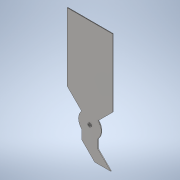
# Autodesk Inventor part: leftside0
Saved by Autodesk Inventor 2020 (Build 240168000, 168)
## iProperties
Created: 2020-04-30
Part Number: leftside0
Material: Generic
Document SubType Name: Modeling
Designer: LENOVO
Density: 1 g/cm^3
Appearance: Default
Author: LENOVO
Autodesk Inventor part; units mm, degrees
ref_plane "YZ Plane" through (0, 0, 0) normal (1, 0, 0) x (0, 1, 0)
ref_plane "XZ Plane" through (0, 0, 0) normal (0, 1, 0) x (-1, 0, 0)
ref_plane "XY Plane" through (0, 0, 0) normal (0, 0, 1) x (1, 0, 0)
sketch "Sketch1" plane through (0, 0, 0) normal (0, 0, 1) x (1, 0, 0)
  line L0 (-100, 150) -> (100, 150)
  line L1 (100, 150) -> (100, -150)
  line L2 (-100, -150) -> (-100, 150)
  line L3 (-100, 150) -> (100, -150) construction
  line L4 (100, 150) -> (-100, -150) construction
  line L5 (100, -150) -> (36.4382, -213.5618)
  line L6 (-35.3571, -283.1536) -> (-35.3571, -323.1554)
  line L7 (-35.3571, -323.1554) -> (21.2114, -379.7239)
  line L8 (35.3571, -283.1536) -> (35.3571, -323.1554)
  line L9 (35.3571, -323.1554) -> (91.9257, -379.7239)
  line L10 (91.9257, -379.7239) -> (21.2114, -379.7239)
  arc A0 (-35.3571, -283.1536) -> (-35.3553, -283.1554) centre (0, -247.8) ccw
  arc A1 (-36.4382, -213.5618) -> (-35.3553, -283.1554) centre (0, -247.8) ccw
  arc A2 (35.3571, -283.1536) -> (36.4382, -213.5618) centre (0, -247.8) ccw
  line L11 (-100, -150) -> (-36.4382, -213.5618)
  point P0 (0, 0)
  point P1 (35.3571, -285.3571)
  constraints: 24 end point, 7 point on circle, 3 centre point, 2 horizontal, 2 midpoint, 1 parallel, 1 perpendicular, 1 point on line, 1 vertical
extrude "Extrusion1" add sketch "Sketch1" along normal blind 3
sketch "Sketch2" plane through (0, 0, 3) normal (0, 0, 1) x (1, 0, 0)
  arc A0 (35.3571, -283.1536) -> (36.4382, -213.5618) centre (0, -247.8) ccw projected
  circle A1 centre (0, -247.8) radius 2.5
  circle A2 centre (0, -247.8) radius 4.75
  circle A3 centre (0, -247.8) radius 7.5
  point P0 (0, 0)
  dimension "d20" = 5
  dimension "d21" = 9.5
  dimension "d22" = 15
  constraints: 3 centre point, 3 coincident
  measures "d20" diameter of A1
  measures "d21" diameter of A2
  measures "d22" diameter of A3
extrude "Extrusion2" cut sketch "Sketch2" against normal blind 3 contours A1
extrude "Extrusion3" add sketch "Sketch2" along normal blind 2 contours A3
body "Solid1"
